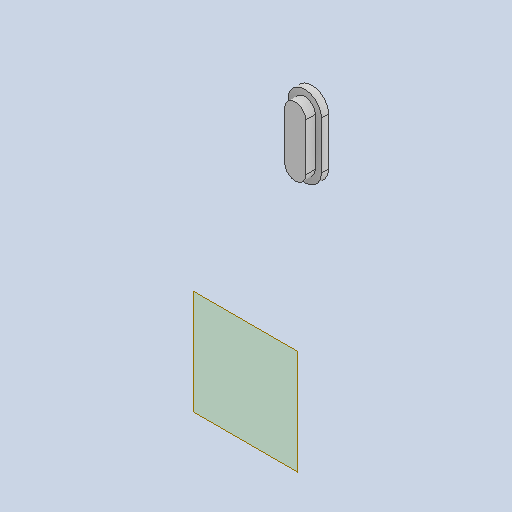
# Autodesk Inventor part: power_button
Saved by Autodesk Inventor 2022 (Build 260153000, 153)
## iProperties
Created: 2022-05-12
Part Number: power_button
Material: Generic
Document SubType Name: Modeling
Designer: simen
Density: 1 g/cm^3
Appearance: Default
Author: simen
## iProperties of the stored document power_button_3DPrint.ipt
Created: 2022-05-12
Part Number: power_button_3DPrint
Material: Generic
Document SubType Name: Modeling
Designer: simen
Density: 1 g/cm^3
Appearance: Default
Author: simen
Autodesk Inventor part; units mm, degrees
ref_plane "YZ Plane" through (0, 0, 0) normal (1, 0, 0) x (0, 1, 0)
ref_plane "XZ Plane" through (0, 0, 0) normal (0, 1, 0) x (-1, 0, 0)
ref_plane "XY Plane" through (0, 0, 0) normal (0, 0, 1) x (1, 0, 0)
ref_plane "Work Plane3" through (0, 1.5, -1.5) normal (0, 0, -1) x (-1, 0, 0)
sketch "Sketch1" plane through (0, 1.5, -1.5) normal (0, 0, -1) x (-1, 0, 0)
  arc A0 (-16, 46) -> (-9, 46) centre (-12.5, 46) ccw
  line L0 (-16, 46) -> (-16, 56)
  arc A1 (-9, 56) -> (-16, 56) centre (-12.5, 56) ccw
  line L1 (-9, 56) -> (-9, 46)
  point P0 (0, -1.5)
  constraints: 4 end point, 4 point on circle, 2 centre point
extrude "Extrusion1" add sketch "Sketch1" along normal blind 1.5
sketch "Sketch2" plane through (0, 1.5, -1.5) normal (0, 0, 1) x (1, 0, 0)
  line L0 (10.3, 56) -> (10.3, 46)
  arc A0 (10.3, 46) -> (14.7, 46) centre (12.5, 46) ccw
  line L1 (14.7, 46) -> (14.7, 56)
  arc A1 (14.7, 56) -> (10.3, 56) centre (12.5, 56) ccw
  point P0 (0, -1.5)
  constraints: 4 end point, 4 point on circle, 2 centre point
extrude "Extrusion2" add sketch "Sketch2" along normal blind 2
body "Solid1"
